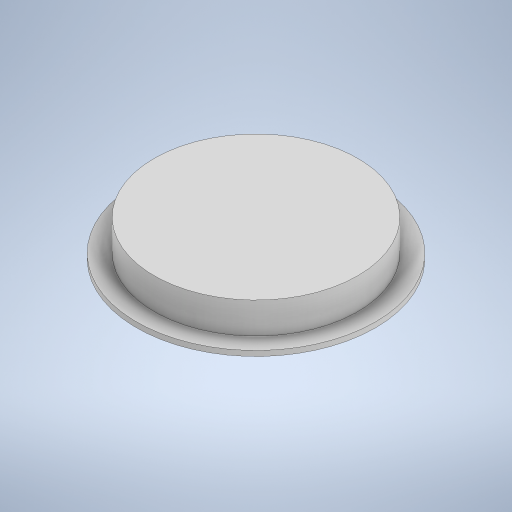
# Autodesk Inventor part: wrist_hone_upper_cover
Saved by Autodesk Inventor 2024.1 (Build 281209000, 209)
## iProperties
Created: 2025-01-23
Part Number: wrist_hone_upper_cover
Material: 一般
Document SubType Name: Modeling
Designer: hibik
Density: 1 g/cm^3
Appearance: 既定
Author: hibik
Autodesk Inventor part; units mm, degrees
ref_plane "YZ Plane" through (0, 0, 0) normal (1, 0, 0) x (0, 1, 0)
ref_plane "XZ Plane" through (0, 0, 0) normal (0, 1, 0) x (-1, 0, 0)
ref_plane "XY Plane" through (0, 0, 0) normal (0, 0, 1) x (1, 0, 0)
sketch "スケッチ1" plane through (0, 0, 0) normal (0, 1, 0) x (-1, 0, 0)
  circle A0 centre (0, 0) radius 9.8
  dimension "d0" = 19.6
  constraints: 1 centre point, 1 coincident
  measures "d0" diameter of A0
extrude "押し出し1" add sketch "スケッチ1" along normal blind 3
sketch "スケッチ2" plane through (0, 0, 0) normal (0, -1, 0) x (1, 0, 0)
  circle A0 centre (-7, 0) radius 3
  circle A1 centre (-7, 0) radius 3.5
  circle A2 centre (0, 0) radius 10
  dimension "d3" = 6
  dimension "d6" = 7
  dimension "d12" = 20
  constraints: 3 centre point, 2 coincident, 1 horizontal alignment, 1 tangent
  measures "d3" diameter of A0
  measures "d6" diameter of A1
  measures "d12" diameter of A2
extrude "押し出し2" add sketch "スケッチ2" along normal blind 3.5 contours A0
extrude "押し出し3" add sketch "スケッチ2" along normal blind 1 contours A2 A1 | A2 A1 picked at (-3.7315, -0.526) picked at (-10.3053, -0.2541)
sketch "スケッチ3" plane through (0, 0, 0) normal (0, -1, 0) x (1, 0, 0)
  circle A0 centre (0, 0) radius 11.5
  dimension "d9" = 23
  constraints: 1 centre point, 1 coincident
  measures "d9" diameter of A0
extrude "押し出し4" add sketch "スケッチ3" along normal blind 0.5
